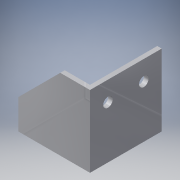
# Autodesk Inventor part: bottom left rail gusset
Saved by Autodesk Inventor 2016 (Build 200138000, 138)
## iProperties
Created: 2016-02-08
Part Number: bottom left rail gusset
Material: Aluminum 6061
Document SubType Name: Modeling
Designer: gus
Density: 2.7 g/cm^3
Appearance: Aluminum - Flat
Mass: 37.8409 g
Surface Area: 99.8985 cm^2
Volume: 14.0151 cm^3
Author: gus
Autodesk Inventor part; units mm, degrees
ref_plane "YZ Plane" through (0, 0, 0) normal (1, 0, 0) x (0, 1, 0)
ref_plane "XZ Plane" through (0, 0, 0) normal (0, 1, 0) x (-1, 0, 0)
ref_plane "XY Plane" through (0, 0, 0) normal (0, 0, 1) x (1, 0, 0)
sketch "Sketch1" plane through (0, 0, 0) normal (0, 0, 1) x (1, 0, 0)
  line L0 (0, 0) -> (0, 21.042)
  line L1 (0, 21.042) -> (29.758, 50.8)
  line L2 (29.758, 50.8) -> (50.8, 50.8)
  line L3 (50.8, 50.8) -> (50.8, 0)
  line L4 (50.8, 0) -> (0, 0)
  dimension "d0" = 50.8
  dimension "d2" = 50.8
  dimension "d3" = 50.8
  dimension "d4" = 135
  constraints: 10 end point, 3 perpendicular, 1 vertical
  measures "d0" distance of L3.end L0.start
  measures "d2" distance of L2.end L3.end
  measures "d3" distance from line of L3.end L1
  measures "d4" angle of L2 L1
extrude "Extrusion1" add sketch "Sketch1" along normal blind 3.175
sketch "Sketch2" plane through (0, 0, 3.175) normal (0, 0, 1) x (1, 0, 0)
  line L0 (50.8, 0) -> (50.8, 50.8) projected
  line L1 (0, 0) -> (50.8, 0) projected
  line L2 (50.8, 50.8) -> (47.625, 50.8)
  line L3 (47.625, 50.8) -> (47.625, 0)
  line L4 (47.625, 0) -> (50.8, 0)
  line L5 (50.8, 0) -> (50.8, 50.8)
  dimension "d7" = 3.175
  constraints: 8 end point, 2 parallel, 1 horizontal, 1 perpendicular, 1 point on line
  measures "d7" distance between parallel lines of L3 L0
extrude "Extrusion2" add sketch "Sketch2" against normal blind 50.8
sketch "Sketch3" plane through (50.8, 0, 3.175) normal (1, 0, 0) x (0, 0, -1)
  circle A0 centre (38.1, 13.8938) radius 3.3734
  circle A1 centre (12.7, 13.8938) radius 3.3734
  line L0 (0, 50.8) -> (50.8, 50.8) projected
  line L1 (0, 0) -> (0, 50.8) projected
  line L2 (0, 0) -> (50.8, 0) projected
  point P0 (3.175, 0)
  dimension "d10" = 6.7469
  dimension "d11" = 6.7469
  dimension "d14" = 12.7
  dimension "d15" = 25.4
  dimension "d25" = 13.8938
  dimension "d26" = 13.8938
  constraints: 2 centre point
  measures "d10" diameter of A0
  measures "d11" diameter of A1
  measures "d14" distance from line of L1 A1.centre
  measures "d15" distance of A0.centre A1.centre
  measures "d25" distance from line of L2 A1.centre
  measures "d26" distance from line of L2 A0.centre
extrude "Extrusion3" cut sketch "Sketch3" against normal blind 3.175
sketch "Sketch5" plane through (0, 0, 0) normal (0, 0, -1) x (-1, 0, 0)
  circle A0 centre (-11.7974, 14.879) radius 3.3734
  circle A1 centre (-29.758, 32.8395) radius 3.3734
  line L0 (0, 21.042) -> (-29.758, 50.8) projected
  line L1 (-29.758, 50.8) -> (-47.7185, 32.8395) construction
  point P0 (0, 0)
  dimension "d27" = 6.7469
  dimension "d28" = 6.7469
  dimension "d29" = 12.7
  dimension "d30" = 12.7
  dimension "d31" = 25.4
  dimension "d32" = 25.4
  dimension "d33" = 12.7
  constraints: 2 centre point, 2 end point, 1 perpendicular
  measures "d27" diameter of A0
  measures "d28" diameter of A1
  measures "d29" distance from line of L0 A0.centre
  measures "d30" distance from line of L0 A1.centre
  measures "d31" distance of A1.centre A0.centre
  measures "d32" distance of L0.end L1.end
  measures "d33" distance from line of L1 A1.centre
extrude "Extrusion5" cut sketch "Sketch5" against normal blind 3.175
body "Solid1"
